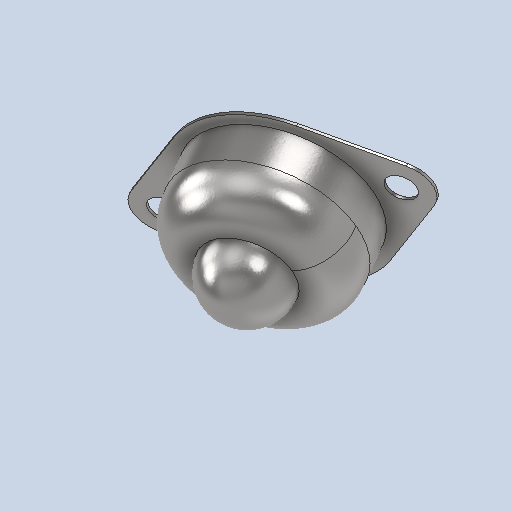
# Autodesk Inventor part: cow_wheel
Saved by Autodesk Inventor 2024 (Build 280153000, 153)
## iProperties
Created: 2024-03-16
Part Number: cow_wheel
Material: 鋼、鍍鋅
Document SubType Name: Modeling
Designer: op04o
Density: 7.85 g/cm^3
Appearance: 鍍鋅
Author: op04o
Autodesk Inventor part; units mm, degrees
ref_plane "YZ Plane" through (0, 0, 0) normal (1, 0, 0) x (0, 1, 0)
ref_plane "XZ Plane" through (0, 0, 0) normal (0, 1, 0) x (-1, 0, 0)
ref_plane "XY Plane" through (0, 0, 0) normal (0, 0, 1) x (1, 0, 0)
sketch "Sketch1" plane through (0, 0, 0) normal (0, 0, 1) x (1, 0, 0)
  circle A0 centre (0, 0) radius 15
  circle A1 centre (0, 0) radius 17
  arc A2 (-23, 4) -> (-25, 0) centre (-20, 0) ccw
  line L0 (-23, 4) -> (-10.2, 13.6)
  circle A3 centre (-19.8, 0) radius 2.5
  line L1 (-25, 0) -> (17, 0)
  circle A4 centre (0, 0) radius 15
  circle A5 centre (0, 0) radius 17
  arc A6 (-25, 0) -> (-23, -4) centre (-20, 0) ccw
  line L2 (-23, -4) -> (-10.2, -13.6)
  circle A7 centre (-19.8, 0) radius 2.5
  line L3 (0, 17) -> (0, -17)
  circle A8 centre (0, 0) radius 15
  circle A9 centre (0, 0) radius 17
  arc A10 (25, 0) -> (23, 4) centre (20, 0) ccw
  line L4 (23, 4) -> (10.2, 13.6)
  circle A11 centre (19.8, 0) radius 2.5
  circle A12 centre (0, 0) radius 15
  circle A13 centre (0, 0) radius 17
  arc A14 (23, -4) -> (25, 0) centre (20, 0) ccw
  line L5 (23, -4) -> (10.2, -13.6)
  circle A15 centre (19.8, 0) radius 2.5
  circle A16 centre (0, 0) radius 7.5
  point P0 (-17, 0)
  dimension "d0" = 30
  dimension "d1" = 34
  dimension "d4" = 5
  dimension "d5" = 25
  dimension "d6" = 5
  dimension "d7" = 19.8
  dimension "d10" = 4
  dimension "d13" = 15
  constraints: 16 centre point, 15 point on circle, 12 end point, 12 symmetric about line, 9 coincident, 2 horizontal alignment, 2 tangent, 1 horizontal, 1 line through centre, 1 vertical, 14 other
  measures "d0" diameter of A0
  measures "d1" diameter of A1
  measures "d4" diameter of A3
  measures "d5" distance of point (0, 0) L1.start
  measures "d6" radius of A2
  measures "d7" distance of point (0, 0) A3.centre
  measures "d10" vertical distance of L1.start L0.start
  measures "d13" diameter of A16
extrude "Extrusion1" add sketch "Sketch1" against normal blind 0.5 contours L1 A16 L3 A0 | L1 A1 L3 A0 | A0 L3 A16 L1 | A0 L3 A1 L1 | L3 A16 L1 A0 | A0 L1 A1 L3 | L3 A1 L1 A0 | A0 L1 A16 L3 | A16 L3 L1 | L1 L3 A16 | A1 L4 A10 A14 L5 | L3 L1 A16 | A16 L1 L3 | L1 A3 A2 L0 A1 | A1 L2 A6 L1 A3
extrude "Extrusion2" add sketch "Sketch1" along normal blind 14 contours L1 A16 L3 A0 | A0 L3 A16 L1 | L3 A16 L1 A0 | A0 L1 A16 L3
extrude "Extrusion3" add sketch "Sketch1" along normal blind 14 contours A16 L3 L1 | L1 L3 A16 | L3 L1 A16 | A16 L1 L3
fillet "Fillet1" radius 7.5 1 edges at (-15, 0, 14) curvature continuous yes
sketch "Sketch2" plane through (0, 0, 14) normal (0, 0, 1) x (1, 0, 0)
  circle A0 centre (0, 0) radius 7.5 construction
  circle A1 centre (0, 0) radius 7.5
  line L0 (-7.5, 0) -> (7.5, 0)
  point P0 (7.5, 0)
  constraints: 2 end point, 1 coincident, 1 horizontal, 1 horizontal alignment, 3 other
revolve "Revolution1" add sketch "Sketch2" angle 360 about axis through (-7.5, 0, 14) along (1, 0, 0) picked at (1.7065, -3.2193) contours A1 L0
body "Solid1"
